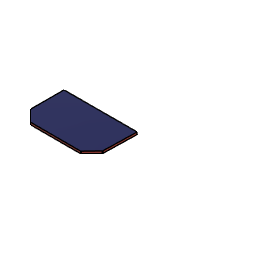
top_cover (Autodesk Fusion 360 design; units mm, degrees)
Autodesk Fusion 360 part; units mm, degrees
sketch "Sketch2" plane through (0, 0, 40) normal (0, 0, 1) x (-1, 0, 0)
  line L0 (-64.9119, -0.1464) -> (0, 0)
  arc A0 (-65.6313, -0.0377) -> (-64.9119, -0.1464) centre (-65.2647, -0.0464) ccw
  line L1 (0, 0) -> (0.0428, 30.0818)
  line L2 (0.0428, 30.0818) -> (-9.9798, 40.1972)
  line L3 (-9.9798, 40.1972) -> (-55.1921, 40.1972)
  line L4 (-55.1921, 40.1972) -> (-64.9187, 30.0818)
  line L5 (-64.9187, 30.0818) -> (-65.6313, -0.0377)
extrude "Extrude2" add sketch "Sketch2" along normal blind 2
sketch "Sketch3" plane through (0, 0, 42) normal (0, 0, 1) x (-1, 0, 0)
  line L0 (-64.9119, -0.1464) -> (0, 0)
  line L1 (-64.9187, 30.0818) -> (-65.6313, -0.0377)
  arc A0 (-65.6313, -0.0377) -> (-64.9119, -0.1464) centre (-65.2647, -0.0464) ccw
  line L2 (0, 0) -> (0.0428, 30.0818)
  line L3 (0.0428, 30.0818) -> (-9.9798, 40.1972)
  line L4 (-9.9798, 40.1972) -> (-55.1921, 40.1972)
  line L5 (-55.1921, 40.1972) -> (-64.9187, 30.0818)
  line L6 (-64.6099, 0.8543) -> (-0.9986, 0.9978)
  line L7 (-0.9986, 0.9978) -> (-0.9578, 29.6708)
  line L8 (-0.9578, 29.6708) -> (-10.3967, 39.1972)
  line L9 (-10.3967, 39.1972) -> (-54.7664, 39.1972)
  line L10 (-54.7664, 39.1972) -> (-63.9282, 29.6691)
  line L11 (-63.9282, 29.6691) -> (-64.6099, 0.8543)
  dimension "d39" = -1
extrude "Extrude3" add sketch "Sketch3" against normal blind 1 contours L6 L7 L8 L9 L10 L11
fillet "Fillet1" radius 0.5 2 edges at (0, 0, 41) (64.9119, 0.1464, 41)
fillet "Fillet2" radius 0.9 4 edges at (64.9187, -30.0818, 41) (55.1921, -40.1972, 41) (9.9798, -40.1972, 41) (-0.0428, -30.0818, 41)
